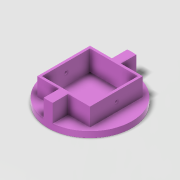
# Autodesk Inventor part: Part6_containter_bottom
Saved by Autodesk Inventor 2020 (Build 240168000, 168)
## iProperties
Created: 2019-07-03
Part Number: Part6_containter_bottom
Material: ABS Plastic
Document SubType Name: Modeling
Designer: kimhos
Density: 1.06 g/cm^3
Appearance: Smooth - Purple
Author: kimhos
Autodesk Inventor part; units mm, degrees
ref_plane "YZ Plane" through (0, 0, 0) normal (1, 0, 0) x (0, 1, 0)
ref_plane "XZ Plane" through (0, 0, 0) normal (0, 1, 0) x (-1, 0, 0)
ref_plane "XY Plane" through (0, 0, 0) normal (0, 0, 1) x (1, 0, 0)
sketch "Sketch2" plane through (0, 0, 0) normal (0, 1, 0) x (-1, 0, 0)
  circle A0 centre (0, 0) radius 14
  circle A1 centre (0, 0) radius 13
  dimension "d0" = 28
  dimension "d110" = 26
  constraints: 2 centre point, 2 coincident
  measures "d0" diameter of A0
  measures "d110" diameter of A1
extrude "Extrusion1" add sketch "Sketch2" along normal blind 2 contours A0 | A1
sketch "Sketch13" plane through (0, 2, 0) normal (0, 1, 0) x (1, 0, 0)
  line L0 (0, 0) -> (8.8, 0)
  line L1 (8.8, 0) -> (8.8, -8.8)
  line L2 (8.8, -8.8) -> (-8.8, -8.8)
  line L3 (-8.8, -8.8) -> (-8.8, 8.8)
  line L4 (-8.8, 8.8) -> (8.8, 8.8)
  line L5 (8.8, 8.8) -> (8.8, 0)
  line L6 (0, 0) -> (8, 0)
  line L7 (8, 0) -> (8, -8)
  line L8 (8, -8) -> (-8, -8)
  line L9 (-8, -8) -> (-8, 8)
  line L10 (-8, 8) -> (8, 8)
  line L11 (8, 8) -> (8, 0)
  line L12 (-8.8, 0) -> (-8, 0)
  dimension "d104" = 8.8
  dimension "d105" = 8.8
  dimension "d106" = 17.6
  dimension "d107" = 17.6
  dimension "d108" = 17.6
  dimension "d109" = 8.8
  dimension "d114" = 8
  dimension "d115" = 8
  dimension "d116" = 16
  dimension "d117" = 16
  dimension "d118" = 16
  dimension "d119" = 8
  constraints: 26 end point, 5 perpendicular, 2 horizontal, 2 midpoint, 2 point on line, 1 parallel, 1 vertical
  measures "d104" distance of L0.start L0.end
  measures "d105" distance of L0.end L1.end
  measures "d106" distance of L1.end L2.end
  measures "d107" distance of L2.end L3.end
  measures "d108" distance of L3.end L4.end
  measures "d109" distance of L4.end L0.end
  measures "d114" distance of L0.start L6.end
  measures "d115" distance of L6.end L7.end
  measures "d116" distance of L7.end L8.end
  measures "d117" distance of L8.end L9.end
  measures "d118" distance of L9.end L10.end
  measures "d119" distance of L10.end L6.end
extrude "Extrusion8" add sketch "Sketch13" along normal blind 6
shell "Shell2" thickness 0.8 removed faces 1 at (-2.9333, 8, -2.9333)
sketch "Sketch14" plane through (-8.8, 2, -8.8) normal (-1, 0, 0) x (0, 0, 1)
  line L0 (17.6, 6) -> (0, 6) projected
  line L1 (8.8, 6) -> (8.8, 3)
  line L2 (8.8, 3) -> (0, 3)
  line L3 (0, 0) -> (0, 6) projected
  circle A0 centre (8.8, 3) radius 0.5
  point P0 (8.8, -2)
  dimension "d121" = 3
  dimension "d122" = 8.8
  dimension "d123" = 1
  constraints: 4 end point, 2 midpoint, 1 centre point, 1 coincident, 1 vertical
  measures "d121" distance of L1.start L1.end
  measures "d122" distance of L1.end L2.end
  measures "d123" diameter of A0
hole "Hole5" at (-8.8, 5, 0) direction (1, 0, 0) diameter 1 depth 20
sketch "Sketch15" plane through (0, 2, 0) normal (0, 1, 0) x (1, 0, 0)
  line L0 (-8.8, -8.8) -> (8.8, -8.8) projected
  circle A0 centre (0, 0) radius 14 projected
  line L1 (0, -8.8) -> (1.5, -8.8)
  line L2 (1.5, -8.8) -> (1.5, -14.8)
  line L3 (1.5, -14.8) -> (-1.5, -14.8)
  line L4 (1.5, -14.8) -> (4.5, -14.8) construction
  line L5 (-1.5, -14.8) -> (-1.5, -8.8)
  line L6 (-1.5, -8.8) -> (1.5, -8.8)
  point P0 (-1.5, -13.9194)
  point P1 (1.5, -13.9194)
  dimension "d132" = 1.5
  dimension "d133" = 6
  dimension "d134" = 3
  dimension "d136" = 6
  dimension "d137" = 3
  constraints: 12 end point, 2 collinear, 2 horizontal, 2 point on line, 1 midpoint, 1 perpendicular
  measures "d132" distance of L1.start L1.end
  measures "d133" distance of L1.end L2.end
  measures "d134" distance of L2.end L3.end
  measures "d136" distance of L3.end L5.end
  measures "d137" distance of L5.end L1.end
extrude "Extrusion9" add sketch "Sketch15" along normal blind 6 contours L0 L2 A0 L5 picked at (0.667, -10.5303)
sketch "Sketch17" plane through (0, 2, 0) normal (0, 1, 0) x (1, 0, 0)
  circle A0 centre (0, 0) radius 14 projected
  line L0 (0, 14) -> (-1.5, 14)
  line L1 (-1.5, 14) -> (-1.5, 8.8)
  line L2 (8.8, 8.8) -> (-8.8, 8.8) projected
  line L3 (-1.5, 8.8) -> (1.5, 8.8)
  line L4 (1.5, 8.8) -> (1.5, 14)
  line L5 (1.5, 14) -> (0, 14)
  point P0 (1.5, 8.8)
  point P1 (1.5, 13.9194)
  point P2 (-1.5, 13.9194)
  dimension "d159" = 1.5
  dimension "d160" = 3
  constraints: 10 end point, 4 perpendicular, 3 horizontal, 2 point on line, 2 other
  measures "d159" distance of L0.start L0.end
  measures "d160" distance of L1.end L3.end
extrude "Extrusion11" add sketch "Sketch17" along normal blind 6 contours L4 L2 L1 A0 picked at (0, 10.5333)
body "Solid1"
